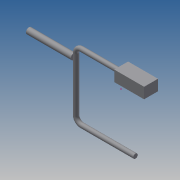
# Autodesk Inventor part: 槓桿
Saved by Autodesk Inventor 2015 (Build 190159000, 159)
## iProperties
Created: 2017-12-28
Part Number: 槓桿
Material: 一般
Document SubType Name: Modeling
Designer: user
Density: 1 g/cm^3
Appearance: 預設
Author: user
Autodesk Inventor part; units mm, degrees
ref_plane "YZ Plane" through (0, 0, 0) normal (1, 0, 0) x (0, 1, 0)
ref_plane "XZ Plane" through (0, 0, 0) normal (0, 1, 0) x (-1, 0, 0)
ref_plane "XY Plane" through (0, 0, 0) normal (0, 0, 1) x (1, 0, 0)
sketch "草圖1" plane through (0, 0, 0) normal (1, 0, 0) x (0, 1, 0)
  circle A0 centre (0, 0) radius 0.75
  dimension "d0" = 1.5
  constraints: 1 centre point, 1 coincident
  measures "d0" diameter of A0
sketch "草圖2" plane through (0, 0, 0) normal (0, 1, 0) x (-1, 0, 0)
  line L0 (0, 0) -> (13.075, 0)
  line L1 (15.075, -2) -> (15.075, -5.0136)
  arc A0 (15.075, -2) -> (13.075, 0) centre (13.075, -2) ccw
  point P0 (15.075, 0)
  dimension "d3" = 2
  constraints: 4 end point, 2 point on circle, 2 point on line, 2 tangent, 1 centre point, 1 horizontal, 1 perpendicular
  measures "d3" radius of A0
sweep "掃掠1" add profiles "草圖1" path "草圖2"
sketch "草圖3" plane through (0, 0, 0) normal (1, 0, 0) x (0, 1, 0)
  line L0 (-2.3279, -1.8091) -> (2.3279, -1.8091)
  line L1 (2.3279, -1.8091) -> (2.3279, 1.8091)
  line L2 (2.3279, 1.8091) -> (-2.3279, 1.8091)
  line L3 (-2.3279, 1.8091) -> (-2.3279, -1.8091)
  line L4 (-2.3279, -1.8091) -> (2.3279, 1.8091) construction
  line L5 (2.3279, -1.8091) -> (-2.3279, 1.8091) construction
  point P0 (0, 0)
  constraints: 12 end point, 2 midpoint, 2 parallel, 1 horizontal, 1 perpendicular
sketch "草圖4" plane through (0, 0, 0) normal (0, 1, 0) x (-1, 0, 0)
  line L0 (15.825, -3.5068) -> (30.825, -3.5068)
  line L1 (30.825, -3.5068) -> (30.825, -2.5068)
  line L2 (30.825, -2.5068) -> (15.825, -2.5068)
  line L3 (15.825, -2.5068) -> (15.825, -3.5068)
  line L4 (15.825, -2) -> (15.825, -5.0136) projected
  point P0 (0, 0)
  point P1 (15.825, -3.0068)
  dimension "d4" = 1
  dimension "d5" = 15
  constraints: 8 end point, 2 midpoint, 2 vertical, 1 horizontal, 1 parallel
  measures "d4" distance of L2.end L0.start
  measures "d5" distance of L1.end L2.end
revolve "迴轉1" add sketch "草圖4" angle 360 about axis through (-15.825, 0, -3.5068) along (-1, 0, 0)
extrude "擠出1" add sketch "草圖3" along normal blind 10
sketch "草圖5" plane through (0, 0, 0) normal (0, 1, 0) x (-1, 0, 0)
  line L0 (14.325, -5.0136) -> (15.825, -5.0136) projected
  line L1 (15.075, -5.0136) -> (15.075, -20.0362)
  line L2 (13.075, -22.0362) -> (-4.7988, -22.0362)
  arc A0 (13.075, -22.0362) -> (15.075, -20.0362) centre (13.075, -20.0362) ccw
  point P0 (0, 0)
  dimension "d9" = 2
  constraints: 4 end point, 2 point on circle, 2 tangent, 1 centre point, 1 midpoint, 1 perpendicular, 1 vertical
  measures "d9" radius of A0
sketch "草圖6" plane through (-15.075, 0, -5.0136) normal (0, 0, -1) x (-1, 0, 0)
  point P0 (-15.075, 0)
sketch "草圖7" plane through (-15.075, 0, -5.0136) normal (0, 0, -1) x (-1, 0, 0)
  circle A0 centre (0, 0) radius 0.75 projected
  point P0 (-15.075, 0)
sweep "掃掠2" add profiles "草圖7" path "草圖5" path curves L1 A0 L2
